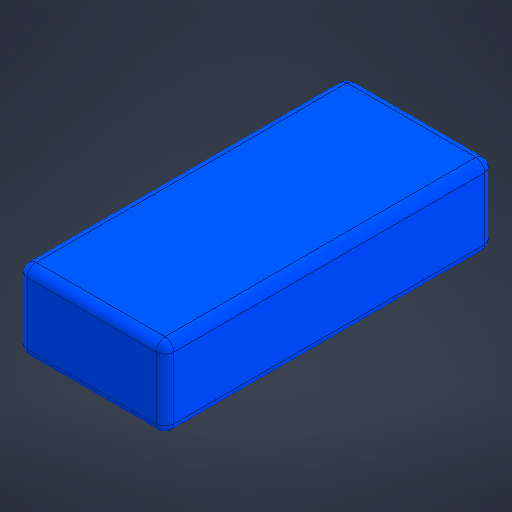
# Autodesk Inventor part: Bateria_2
Saved by Autodesk Inventor 2026.1 (Build 301233020, 233B)
## iProperties
Created: 2026-02-10
Part Number: Bateria_2
Material: Genérico
Document SubType Name: Modeling
Designer: celio
Density: 1 g/cm^3
Appearance: Padrão
Author: celio
Autodesk Inventor part; units mm, degrees
ref_plane "YZ Plane" through (0, 0, 0) normal (1, 0, 0) x (0, 1, 0)
ref_plane "XZ Plane" through (0, 0, 0) normal (0, 1, 0) x (-1, 0, 0)
ref_plane "XY Plane" through (0, 0, 0) normal (0, 0, 1) x (1, 0, 0)
sketch "Esboço1" plane through (0, 0, 0) normal (0, 1, 0) x (-1, 0, 0)
  line L0 (-16.5, 37) -> (16.5, 37)
  line L1 (16.5, 37) -> (16.5, -37)
  line L2 (16.5, -37) -> (-16.5, -37)
  line L3 (-16.5, -37) -> (-16.5, 37)
  line L4 (-16.5, 37) -> (16.5, -37) construction
  line L5 (16.5, 37) -> (-16.5, -37) construction
  point P0 (0, 0)
  dimension "d0" = 33
  dimension "d1" = 74
  constraints: 12 end point, 2 midpoint, 2 parallel, 1 horizontal, 1 perpendicular
  measures "d0" distance of L1.end L2.end
  measures "d1" distance of L0.end L1.end
extrude "Extrusão1" add sketch "Esboço1" along normal blind 18
fillet "Arredondamento1" radius 2 12 edges at (16.5, 18, 0) (0, 18, 37) (-16.5, 18, 0) (0, 18, -37) (-16.5, 0, 0) (-16.5, 9, 37) (0, 0, 37) (16.5, 9, 37) (16.5, 0, 0) (0, 0, -37) (16.5, 9, -37) (-16.5, 9, -37)
